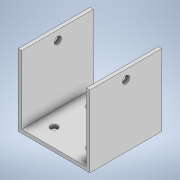
# Autodesk Inventor part: blaket_1
Saved by Autodesk Inventor 2021.4 (Build 254397000, 397)
## iProperties
Created: 2023-10-13
Part Number: blaket_1
Material: 一般
Document SubType Name: Modeling
Designer: ryusei
Density: 1 g/cm^3
Appearance: 既定
Author: ryusei
Autodesk Inventor part; units mm, degrees
ref_plane "YZ Plane" through (0, 0, 0) normal (1, 0, 0) x (0, 1, 0)
ref_plane "XZ Plane" through (0, 0, 0) normal (0, 1, 0) x (-1, 0, 0)
ref_plane "XY Plane" through (0, 0, 0) normal (0, 0, 1) x (1, 0, 0)
sketch "スケッチ1" plane through (0, 0, 0) normal (0, 1, 0) x (-1, 0, 0)
  line L0 (20, 20) -> (-20, 20)
  line L1 (-20, 20) -> (-20, -20)
  line L2 (-20, -20) -> (20, -20)
  line L3 (20, -20) -> (20, 20)
  line L4 (20, 20) -> (-20, -20) construction
  line L5 (-20, 20) -> (20, -20) construction
  point P0 (0, 0)
  dimension "d0" = 40
  dimension "d1" = 40
  constraints: 12 end point, 2 midpoint, 2 parallel, 1 horizontal, 1 perpendicular
  measures "d0" distance of L2.end L1.end
  measures "d1" distance of L1.end L0.end
extrude "押し出し1" add sketch "スケッチ1" along normal blind 40
sketch "スケッチ2" plane through (0, 40, 0) normal (0, 1, 0) x (1, 0, 0)
  line L0 (20, 20) -> (-20, 20) projected
  line L1 (-18, -20) -> (18, -20)
  line L2 (18, -20) -> (18, 20)
  line L3 (18, 20) -> (-18, 20)
  line L4 (-18, 20) -> (-18, -20)
  line L5 (-18, -20) -> (18, 20) construction
  line L6 (18, -20) -> (-18, 20) construction
  point P0 (0, 0)
  dimension "d4" = 36
  constraints: 12 end point, 2 midpoint, 2 parallel, 1 horizontal, 1 perpendicular, 1 point on line
  measures "d4" distance of L3.end L2.end
extrude "押し出し2" cut sketch "スケッチ2" against normal blind 38
sketch "スケッチ3" plane through (0, 0, 0) normal (0, -1, 0) x (1, 0, 0)
  line L0 (-20, 20) -> (20, 20) projected
  line L1 (20, 20) -> (20, -20) projected
  point P0 (0, 0)
  point P1 (10, 10)
  point P2 (10, -10)
  point P3 (-10, 10)
  point P4 (-10, -10)
  dimension "d7" = 10
  dimension "d8" = 10
  dimension "d11" = 20
  dimension "d14" = 20
  constraints: 1 horizontal, 1 vertical, 3 other
  measures "d7" distance from line of L0 point (10, 10)
  measures "d8" distance from line of L1 point (10, 10)
  measures "d11" distance of point (10, 10) point (10, -10)
  measures "d14" distance of point (10, 10) point (-10, 10)
hole "穴1" at (10, 0, 10) at (10, 0, -10) at (-10, 0, 10) at (-10, 0, -10) direction (0, 1, 0) diameter 4 end through all
sketch "スケッチ4" plane through (20, 0, 20) normal (1, 0, 0) x (0, 0, -1)
  line L0 (0, 40) -> (40, 40) projected
  line L1 (0, 0) -> (0, 40) projected
  point P0 (20, 0)
  point P1 (20, 35)
  dimension "d24" = 5
  dimension "d25" = 20
  measures "d24" distance from line of L0 point (20, 35)
  measures "d25" distance from line of L1 point (20, 35)
hole "穴2" at (20, 35, 0) direction (-1, 0, 0) diameter 4 end through all
